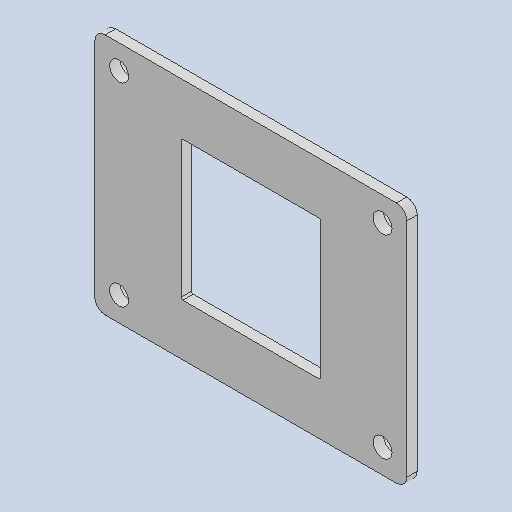
# Autodesk Inventor part: NDV-3001 Branch flange 01
Saved by Autodesk Inventor 2026.2 (Build 302298000, 298)
## iProperties
Created: 2026-10-05
Part Number: NDV-3001 Branch flange 01
Material: Generic
Document SubType Name: Sheet Metal
Designer: admin
Density: 1 g/cm^3
Sheet Metal Rule: Default_mm
Appearance: Default
Stock Number: Фланец луча
Flat Pattern Width: 7 cm
Flat Pattern Length: 9 cm
Flat Pattern Area: 63 cm^2
Sheet Metal Width: 70,000 mm
Sheet Metal Length: 90,000 mm
Sheet Metal Area: 6300,000 mm^2
Author: admin
Autodesk Inventor part; units mm, degrees
ref_plane "YZ Plane" through (0, 0, 0) normal (1, 0, 0) x (0, 1, 0)
ref_plane "XZ Plane" through (0, 0, 0) normal (0, 1, 0) x (-1, 0, 0)
ref_plane "XY Plane" through (0, 0, 0) normal (0, 0, 1) x (1, 0, 0)
derived "NDV-0010 Parameters 01.ipt"
sketch "sk_flange" plane through (0, 0, 0) normal (0, 0, 1) x (1, 0, 0)
  line L0 (-45, -35) -> (45, -35)
  line L1 (45, -35) -> (45, 35)
  line L2 (45, 35) -> (-45, 35)
  line L3 (-45, 35) -> (-45, -35)
  line L4 (-45, -35) -> (45, 35) construction
  line L5 (45, -35) -> (-45, 35) construction
  line L6 (-20.1, -20.1) -> (20.1, -20.1)
  line L7 (20.1, -20.1) -> (20.1, 20.1)
  line L8 (20.1, 20.1) -> (-20.1, 20.1)
  line L9 (-20.1, 20.1) -> (-20.1, -20.1)
  line L10 (-20.1, -20.1) -> (20.1, 20.1) construction
  line L11 (20.1, -20.1) -> (-20.1, 20.1) construction
  circle A0 centre (38, 28) radius 2.75
  circle A1 centre (38, -28) radius 2.75
  circle A2 centre (-38, 28) radius 2.75
  circle A3 centre (-38, -28) radius 2.75
  point P0 (0, 0)
  dimension "d1" = 90
  dimension "d2" = 70
  dimension "d3" = 40.2
  dimension "d4" = 40.2
  dimension "d5" = 5.5
  dimension "d6" = 38
  dimension "d7" = 28
  dimension "d8" = 5.5
  dimension "d9" = 38
  dimension "d10" = 28
  dimension "d11" = 5.5
  dimension "d12" = 38
  dimension "d13" = 28
  dimension "d14" = 5.5
  dimension "d15" = 38
  dimension "d16" = 28
  measures "d1" distance of L0.start L0.end
  measures "d2" distance of L0.end L1.end
  measures "d3" distance of L6.start L6.end
  measures "d4" distance of L6.end L7.end
  measures "d5" diameter of A0
  measures "d6" horizontal distance of point (0, 0) A0.centre
  measures "d7" vertical distance of point (0, 0) A0.centre
  measures "d8" diameter of A1
  measures "d9" horizontal distance of point (0, 0) A1.centre
  measures "d10" vertical distance of point (0, 0) A1.centre
  measures "d11" diameter of A2
  measures "d12" horizontal distance of point (0, 0) A2.centre
  measures "d13" vertical distance of point (0, 0) A2.centre
  measures "d14" diameter of A3
  measures "d15" horizontal distance of point (0, 0) A3.centre
  measures "d16" vertical distance of point (0, 0) A3.centre
extrude "Plate1" add sketch "sk_flange" along normal blind 3
fillet "Corner Round1" radius 3 4 edges at (-45, 35, 1.5) (-45, -35, 1.5) (45, 35, 1.5) (45, -35, 1.5)
fillet "Corner Round2" radius 0.5 4 edges at (-20.1, -20.1, 1.5) (-20.1, 20.1, 1.5) (20.1, 20.1, 1.5) (20.1, -20.1, 1.5)
equation "\"d1\" = Flange_W"
equation "\"d2\" = Flange_H"
equation "\"d3\" = Flange_hole"
equation "\"d4\" = Flange_hole"
equation "\"d5\" = Rivet_hole"
equation "\"d6\" = 0.5 * Flange_pitch_h"
equation "\"d7\" = 0.5 * Flange_pitch_v"
equation "\"d8\" = Rivet_hole"
equation "\"d9\" = 0.5 * Flange_pitch_h"
equation "\"d10\" = 0.5 * Flange_pitch_v"
equation "\"d11\" = Rivet_hole"
equation "\"d12\" = 0.5 * Flange_pitch_h"
equation "\"d13\" = 0.5 * Flange_pitch_v"
equation "\"d14\" = Rivet_hole"
equation "\"d15\" = 0.5 * Flange_pitch_h"
equation "\"d16\" = 0.5 * Flange_pitch_v"
equation "\"d18\" = Flange_corner_R"
equation "\"d19\" = Flange_hole_corner_R"
equation "\"d17\" = Thickness"
equation "\"Thickness\" = Flange_thickness"
equation "\"BendRadius\" = Thickness"
equation "\"BendReliefWidth\" = Thickness"
equation "\"BendReliefDepth\" = 0.5 * Thickness"
equation "\"CornerReliefSize\" = 4 * Thickness"
equation "\"MinimumRemnant\" = 2 * Thickness"
equation "\"TransitionRadius\" = BendRadius"
equation "\"JacobiRadiusSize\" = BendRadius"
equation "\"GapSize\" = Thickness"
equation "\"Flange_W\" = 90"
equation "\"Flange_H\" = 70"
equation "\"Flange_hole\" = 40.2"
equation "\"Rivet_hole\" = 5.5"
equation "\"Flange_corner_R\" = 3"
equation "\"Flange_hole_corner_R\" = 0.5"
equation "\"Flange_thickness\" = 3"
equation "\"Flange_pitch_h\" = 76"
equation "\"Flange_pitch_v\" = 56"
body "Solid1"
